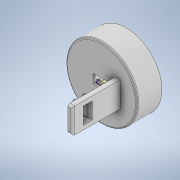
# Autodesk Inventor part: Base
Saved by Autodesk Inventor 2020 (Build 240168000, 168)
## iProperties
Created: 2020-02-27
Part Number: Base
Material: Generic
Document SubType Name: Modeling
Designer: othscs164
Density: 1 g/cm^3
Appearance: Default
Author: othscs164
Autodesk Inventor part; units mm, degrees
ref_plane "YZ Plane" through (0, 0, 0) normal (1, 0, 0) x (0, 1, 0)
ref_plane "XZ Plane" through (0, 0, 0) normal (0, 1, 0) x (-1, 0, 0)
ref_plane "XY Plane" through (0, 0, 0) normal (0, 0, 1) x (1, 0, 0)
sketch "Sketch1" plane through (0, 0, 0) normal (0, 0, 1) x (1, 0, 0)
  circle A0 centre (0, 0) radius 41.275
  circle A1 centre (0, 0) radius 47.625
  dimension "d0" = 82.55
  dimension "d1" = 6.35
  constraints: 2 centre point, 1 coincident
  measures "d0" diameter of A0
  measures "d1" radial gap between concentric circles of A0 A1
extrude "Extrusion1" add sketch "Sketch1" along normal blind 25.4
sketch "Sketch2" plane through (0, 0, 25.4) normal (0, 0, 1) x (1, 0, 0)
  circle A0 centre (0, 0) radius 47.625
  constraints: 1 centre point, 1 coincident
extrude "Extrusion2" add sketch "Sketch2" along normal blind 3.175
sketch "Sketch3" plane through (0, 0, 25.4) normal (0, 0, -1) x (-1, 0, 0)
  line L0 (11, 6) -> (-11, 6)
  line L1 (-11, 6) -> (-11, -6)
  line L2 (-11, -6) -> (11, -6)
  line L3 (11, -6) -> (11, 6)
  line L4 (11, 6) -> (-11, -6) construction
  line L5 (-11, 6) -> (11, -6) construction
  line L6 (-10.6662, 8.8412) -> (10.6662, 8.8412)
  line L7 (13.8412, 5.6662) -> (13.8412, -5.6662)
  line L8 (10.6662, -8.8412) -> (-10.6662, -8.8412)
  line L9 (-13.8412, -5.6662) -> (-13.8412, 5.6662)
  arc A0 (-10.6662, 8.8412) -> (-13.8412, 5.6662) centre (-10.6662, 5.6662) ccw
  arc A1 (-13.8412, -5.6662) -> (-10.6662, -8.8412) centre (-10.6662, -5.6662) ccw
  arc A2 (10.6662, -8.8412) -> (13.8412, -5.6662) centre (10.6662, -5.6662) ccw
  arc A3 (13.8412, 5.6662) -> (10.6662, 8.8412) centre (10.6662, 5.6662) ccw
  point P0 (0, 0)
  dimension "d6" = 22
  dimension "d7" = 12
  dimension "d8" = 3.175
  constraints: 20 end point, 8 point on circle, 8 tangent, 4 centre point, 4 parallel, 3 equal radius, 2 midpoint, 2 perpendicular, 1 horizontal, 3 other
  measures "d6" distance of L2.end L1.end
  measures "d7" distance of L1.end L0.end
  measures "d8" radius of A0
extrude "Extrusion3" add sketch "Sketch3" along normal blind 6.35
chamfer "Chamfer1" distance 1.5875 angle 45 8 edges at (0, 8.8412, 19.05) (12.9113, 7.9113, 19.05) (13.8412, 0, 19.05) (12.9113, -7.9113, 19.05) (0, -8.8412, 19.05) (-12.9113, -7.9113, 19.05) (-13.8412, 0, 19.05) (-12.9113, 7.9113, 19.05)
sketch "Sketch5" plane through (-13.8412, -5.6662, 25.4) normal (-1, 0, 0) x (0, 0, 1)
  line L0 (-0.1094, 0) -> (-8.0486, 0)
  line L1 (-8.0486, 0) -> (-8.0486, 11.3324)
  line L2 (-8.0486, 11.3324) -> (-0.1094, 11.3324)
  line L3 (-0.1094, 11.3324) -> (-0.1094, 0)
  point P0 (-25.4, 5.6662)
  constraints: 8 end point, 2 parallel, 1 horizontal, 1 perpendicular
extrude "Extrusion5" cut sketch "Sketch5" against normal blind 28.575
sketch "Sketch6" plane through (0, 0, 0) normal (0, 0, -1) x (-1, 0, 0)
  circle A0 centre (0, 0) radius 47.625 projected
  circle A1 centre (0, 0) radius 41.275 projected
extrude "Extrusion6" add sketch "Sketch6" along normal blind 4.5
chamfer "Chamfer2" distance 1.5875 angle 45 1 edges at (-47.625, 0, 28.575)
fillet "Fillet2" radius 1.5875 1 edges at (-46.0375, 0, 28.575)
fillet "Fillet3" radius 1.5875 1 edges at (-47.625, 0, 26.9875)
sketch "Sketch7" plane through (0, 0, 25.4) normal (0, 0, -1) x (-1, 0, 0)
  circle A0 centre (0, 0) radius 41.275 projected
  line L0 (-10.6662, 8.8412) -> (10.6662, 8.8412) projected
  arc A1 (13.8412, 5.6662) -> (10.6662, 8.8412) centre (10.6662, 5.6662) ccw projected
  line L1 (13.8412, 5.6662) -> (13.8412, -5.6662) projected
  arc A2 (10.6662, -8.8412) -> (13.8412, -5.6662) centre (10.6662, -5.6662) ccw projected
  line L2 (10.6662, -8.8412) -> (-10.6662, -8.8412) projected
  arc A3 (-13.8412, -5.6662) -> (-10.6662, -8.8412) centre (-10.6662, -5.6662) ccw projected
  line L3 (-13.8412, -5.6662) -> (-13.8412, 5.6662) projected
  arc A4 (-10.6662, 8.8412) -> (-13.8412, 5.6662) centre (-10.6662, 5.6662) ccw projected
  line L4 (10.6662, 7.2537) -> (10.6662, 8.8412) projected
  arc A5 (12.2537, 5.6662) -> (10.6662, 7.2537) centre (10.6662, 5.6662) ccw projected
  line L5 (13.8412, 5.6662) -> (12.2537, 5.6662) projected
  arc A6 (13.8412, 5.6662) -> (10.6662, 8.8412) centre (10.6662, 5.6662) ccw projected
  line L6 (-10.6662, 7.2537) -> (10.6662, 7.2537) projected
  line L7 (-12.2537, 5.6662) -> (-11, 5.6662) projected
  line L8 (-11, 5.6662) -> (-11, 6) projected
  line L9 (-11, 6) -> (11, 6) projected
  line L10 (11, 6) -> (11, 5.6662) projected
  line L11 (11, 5.6662) -> (12.2537, 5.6662) projected
  arc A7 (12.2537, 5.6662) -> (10.6662, 7.2537) centre (10.6662, 5.6662) ccw projected
  line L12 (-10.6662, 7.2537) -> (10.6662, 7.2537) projected
  arc A8 (-10.6662, 7.2537) -> (-12.2537, 5.6662) centre (-10.6662, 5.6662) ccw projected
  line L13 (-10.6662, 8.8412) -> (-10.6662, 7.2537) projected
  line L14 (-10.6662, 7.2537) -> (10.6662, 7.2537) projected
  line L15 (10.6662, 7.2537) -> (10.6662, 8.8412) projected
  line L16 (10.6662, 8.8412) -> (-10.6662, 8.8412) projected
  line L17 (-11, 6) -> (11, 6) projected
  line L18 (10.6662, 8.8412) -> (-10.6662, 8.8412) projected
  line L19 (11, 5.6662) -> (12.2537, 5.6662) projected
  line L20 (10.6662, 8.8412) -> (-10.6662, 8.8412)
  line L21 (-10.6662, -8.8412) -> (10.6662, -8.8412) projected
  line L22 (10.6662, -8.8412) -> (-10.6662, -8.8412)
  arc A9 (13.8412, 5.6662) -> (10.6662, 8.8412) centre (10.6662, 5.6662) ccw projected
  arc A10 (13.8412, 5.6662) -> (10.6662, 8.8412) centre (10.6662, 5.6662) ccw
  line L23 (10.6662, -8.8412) -> (10.6662, -7.2537) projected
  arc A11 (10.6662, -8.8412) -> (13.8412, -5.6662) centre (10.6662, -5.6662) ccw
  arc A12 (-13.8412, -5.6662) -> (-10.6662, -8.8412) centre (-10.6662, -5.6662) ccw
  arc A13 (-10.6662, 8.8412) -> (-13.8412, 5.6662) centre (-10.6662, 5.6662) ccw projected
  arc A14 (-10.6662, 8.8412) -> (-13.8412, 5.6662) centre (-10.6662, 5.6662) ccw
  line L24 (11, -6) -> (11, 6) projected
  line L25 (11, 5.6662) -> (11, 6)
  line L26 (11, 6) -> (-11, 6)
  line L27 (-11, 5.6662) -> (-11, -5.6662) projected
  line L28 (-11, 6) -> (-11, 5.6662)
  line L29 (-11, 5.6662) -> (-13.8412, 5.6662)
  line L30 (-11, -5.6662) -> (-13.8412, -5.6662) projected
  line L31 (-13.8412, -5.6662) -> (-11, -5.6662)
  line L32 (-11, -6) -> (-11, -5.6662) projected
  line L33 (-11, -5.6662) -> (-11, -6)
  line L34 (-11, -6) -> (11, -6)
  line L35 (11, -5.6662) -> (11, -6) projected
  line L36 (11, -6) -> (11, -5.6662)
  line L37 (13.8412, -5.6662) -> (11, -5.6662) projected
  line L38 (11, -5.6662) -> (13.8412, -5.6662)
  line L39 (10.6662, 7.2537) -> (10.6662, 8.8412) projected
  arc A15 (13.8412, 5.6662) -> (10.6662, 8.8412) centre (10.6662, 5.6662) ccw
  arc A16 (-10.6662, 8.8412) -> (-13.8412, 5.6662) centre (-10.6662, 5.6662) ccw
  line L40 (10.6662, 8.8412) -> (-10.6662, 8.8412)
  line L41 (11, 6) -> (-11, 6)
  line L42 (-11, 5.6662) -> (-11, 6)
  line L43 (-13.8412, 5.6662) -> (-12.2537, 5.6662) projected
  line L44 (-11, 5.6662) -> (-13.8412, 5.6662)
  line L45 (13.8412, 5.6662) -> (13.8412, -5.6662) projected
  line L46 (13.8412, 5.6662) -> (11, 5.6662)
  constraints: 32 end point, 13 point on circle, 6 centre point, 6 perpendicular, 4 collinear, 4 tangent, 2 concentric, 2 horizontal, 2 point on line, 2 vertical, 1 parallel
sketch "Sketch8" plane through (0, 0, 28.575) normal (0, 0, 1) x (1, 0, 0)
  line L0 (0, 0) -> (18.6341, 0)
  line L1 (18.6341, 0) -> (18.6341, -16.7894)
  line L2 (18.6341, -16.7894) -> (18.6341, 0)
  line L3 (18.6341, 0) -> (18.6341, 16.7894)
  line L4 (18.6341, 16.7894) -> (24.9841, 16.7894)
  line L5 (24.9841, 16.7894) -> (24.9841, -16.7894)
  line L6 (24.9841, -16.7894) -> (18.6341, -16.7894)
  dimension "d28" = 16.7894
  dimension "d29" = 6.35
  dimension "d30" = 33.5788
  constraints: 14 end point, 5 perpendicular, 1 horizontal, 1 point on line
  measures "d28" distance of L0.end L3.end
  measures "d29" distance of L3.end L4.end
  measures "d30" distance of L4.end L5.end
extrude "Extrusion7" add sketch "Sketch8" along normal blind 63.5
fillet "Fillet4" radius 3.175 3 edges at (24.9841, 0, 92.075) (21.8091, -16.7894, 92.075) (21.8091, 16.7894, 92.075)
sketch "Sketch9" plane through (18.6341, -16.7894, 28.575) normal (-1, 0, 0) x (0, 0, 1)
  line L0 (34.3149, 27.4309) -> (34.3745, 6.0985)
  line L1 (51.9973, 27.4803) -> (52.0568, 6.1479)
  arc A0 (37.481, 30.6147) -> (34.3149, 27.4309) centre (37.4899, 27.4398) ccw
  arc A1 (51.9973, 27.4803) -> (48.8134, 30.6464) centre (48.8223, 27.4714) ccw
  arc A2 (48.8907, 2.9641) -> (52.0568, 6.1479) centre (48.8818, 6.139) ccw
  arc A3 (34.3745, 6.0985) -> (37.5583, 2.9324) centre (37.5494, 6.1074) ccw
  line L2 (37.4889, 27.7735) -> (37.1552, 27.7726)
  line L3 (37.1552, 27.7726) -> (37.2166, 5.7727)
  line L4 (37.2166, 5.7727) -> (37.5504, 5.7736)
  line L5 (37.5504, 5.7736) -> (37.5583, 2.9324)
  line L6 (48.8907, 2.9641) -> (48.8828, 5.8053)
  line L7 (48.8828, 5.8053) -> (49.2166, 5.8062)
  line L8 (49.2166, 5.8062) -> (49.1551, 27.8061)
  line L9 (49.1551, 27.8061) -> (48.8213, 27.8052)
  line L10 (48.8213, 27.8052) -> (48.8134, 30.6464)
  arc A4 (37.481, 30.6147) -> (34.3149, 27.4309) centre (37.4899, 27.4398) ccw
  arc A5 (34.3745, 6.0985) -> (37.5583, 2.9324) centre (37.5494, 6.1074) ccw
  line L11 (34.3149, 27.4309) -> (34.3745, 6.0985)
  line L12 (37.1552, 27.7726) -> (37.2166, 5.7727)
  line L13 (37.5504, 5.7736) -> (37.2166, 5.7727)
  line L14 (37.5504, 5.7736) -> (37.5583, 2.9324)
  line L15 (37.481, 30.6147) -> (37.4889, 27.7735)
  line L16 (48.8134, 30.6464) -> (37.5583, 2.9324)
  line L17 (52.027, 16.8141) -> (34.3447, 16.7647)
  line L18 (0, 0) -> (0, 33.5788) projected
  line L19 (43.1859, 16.7894) -> (43.1472, 30.6306)
  line L20 (0, 0) -> (60.325, 0) projected
  line L21 (63.5, 30.4038) -> (63.5, 3.175) projected
  line L22 (63.5, 16.7894) -> (-3.2844, 16.7894)
  line L23 (-3.2844, 22.4556) -> (-3.2844, 11.1232) projected
  line L24 (30.1078, 16.7894) -> (30.1078, 22.4556)
  point P0 (-28.575, 16.7894)
  point P1 (37.5583, 2.9324)
  point P2 (37.481, 30.6147)
  point P3 (34.3149, 27.4309)
  point P4 (34.3446, 16.7894)
  point P5 (37.1858, 16.7894)
  point P6 (37.1859, 16.7726)
  point P7 (49.1858, 16.8062)
  point P8 (52.0271, 16.7894)
  point P9 (49.1859, 16.7894)
  constraints: 40 end point, 12 point on circle, 6 centre point, 6 midpoint, 5 perpendicular, 2 concentric, 1 point on line, 1 tangent, 1 vertical, 4 other
extrude "Extrusion8" add sketch "Sketch9" along normal blind 6.35 contours L17 L3 L4 L5 A3 L0 | L0 A0 L15 L2 L3 L22 | A1 L1 L17 L8 L9 L10 | L22 L1 A2 L6 L7 L8
chamfer "Chamfer3" distance 1.5875 angle 45 8 edges at (12.2841, -5.3207, 80.617) (12.2841, -12.8891, 79.7082) (12.2841, 5.3578, 80.5871) (12.2841, 12.9333, 79.6361) (12.2841, 5.3207, 62.9047) (12.2841, 12.8891, 63.8136) (12.2841, -12.9333, 63.8857) (12.2841, -5.3578, 62.9346)
sketch "Sketch10" plane through (0, 0, 25.4) normal (0, 0, -1) x (-1, 0, 0)
  line L0 (11, 6) -> (-11, 6) projected
  line L1 (-11, -6) -> (11, -6) projected
  line L2 (-11, 6) -> (11, 6)
  line L3 (11, 6) -> (11, -6)
  line L4 (11, -6) -> (-11, -6)
  line L5 (-11, -6) -> (-11, 6)
  point P0 (0, 0)
  constraints: 8 end point, 2 parallel, 1 horizontal, 1 perpendicular
extrude "Extrusion9" cut sketch "Sketch10" against normal up to surface (3.175 mm away)
sketch "Sketch11" plane through (18.6341, -16.7894, 28.575) normal (-1, 0, 0) x (0, 0, 1)
  line L0 (48.8213, 27.8052) -> (49.1551, 27.8061) projected
  line L1 (37.2166, 5.7727) -> (37.1859, 16.7726) projected
  line L2 (49.1551, 27.8061) -> (37.2166, 27.8061)
  line L3 (37.2166, 27.8061) -> (37.2166, 5.7727)
  line L4 (37.2166, 5.7727) -> (49.1551, 5.7727)
  line L5 (49.1551, 5.7727) -> (49.1551, 27.8061)
  point P0 (-28.575, 16.7894)
  constraints: 8 end point, 2 parallel, 1 horizontal, 1 perpendicular
extrude "Extrusion10" cut sketch "Sketch11" against normal up to surface (6.35 mm away)
body "Solid1"
